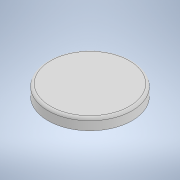
# Autodesk Inventor part: lid-v1
Saved by Autodesk Inventor 2022 (Build 260153000, 153)
## iProperties
Created: 2021-07-14
Part Number: lid-v1
Material: Generic
Document SubType Name: Modeling
Designer: dncob
Density: 1 g/cm^3
Appearance: Default
Author: dncob
Autodesk Inventor part; units mm, degrees
ref_plane "YZ Plane" through (0, 0, 0) normal (1, 0, 0) x (0, 1, 0)
ref_plane "XZ Plane" through (0, 0, 0) normal (0, 1, 0) x (-1, 0, 0)
ref_plane "XY Plane" through (0, 0, 0) normal (0, 0, 1) x (1, 0, 0)
sketch "Sketch2" plane through (0, 0, 0) normal (0, 0, 1) x (1, 0, 0)
  line L0 (0, 0) -> (48.55, 0)
  line L1 (48.55, 0) -> (48.55, -13)
  line L2 (48.55, -13) -> (44.55, -13)
  line L3 (44.55, -13) -> (44.55, -4)
  line L4 (44.55, -4) -> (38.55, -4)
  line L5 (38.55, -4) -> (38.55, -7)
  line L6 (38.55, -7) -> (0, -7)
  line L7 (0, -7) -> (0, 0)
  dimension "d0" = 48.55
  dimension "d1" = 4
  dimension "d2" = 6
  dimension "d3" = 13
  dimension "d4" = 4
  dimension "d5" = 7
  constraints: 16 end point, 6 perpendicular, 1 horizontal, 1 vertical
  measures "d0" distance of L0.start L0.end
  measures "d1" distance of L1.end L2.end
  measures "d2" distance of L3.end L4.end
  measures "d3" distance of L0.end L1.end
  measures "d4" distance between parallel lines of L4 L0
  measures "d5" distance between parallel lines of L6 L0
revolve "Revolution1" add sketch "Sketch2" angle 360 about axis through (0, -7, 0) along (0, 1, 0)
fillet "Fillet1" radius 3 1 edges at (-48.55, 0, 0)
sketch "Sketch3" plane through (0, -7, 0) normal (0, -1, 0) x (1, 0, 0)
  circle A0 centre (0, -19.55) radius 17
  circle A1 centre (0, 0) radius 38.55 projected
  circle A2 centre (0, 19.55) radius 17
  dimension "d8" = 34
  dimension "d11" = 360
  dimension "d15" = 19.55
  constraints: 2 centre point, 1 vertical alignment, 5 other
  measures "d8" diameter of A0
  measures "d15" distance of A0.centre point (0, 0)
extrude "Extrusion1" cut sketch "Sketch3" against normal blind 5 contours A0 | A2
body "Solid1"
